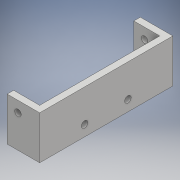
# Autodesk Inventor part: Część2
Saved by Autodesk Inventor 2017 (Build 210142000, 142)
## iProperties
Created: 2019-10-20
Part Number: Część2
Material: Ogólny
Document SubType Name: Modeling
Designer: patry
Density: 1 g/cm^3
Appearance: Domyślna
Author: patry
Autodesk Inventor part; units mm, degrees
ref_plane "YZ Plane" through (0, 0, 0) normal (1, 0, 0) x (0, 1, 0)
ref_plane "XZ Plane" through (0, 0, 0) normal (0, 1, 0) x (-1, 0, 0)
ref_plane "XY Plane" through (0, 0, 0) normal (0, 0, 1) x (1, 0, 0)
sketch "Szkic1" plane through (0, 0, 0) normal (0, 1, 0) x (-1, 0, 0)
  line L0 (7, -35.6103) -> (-8, -35.6103)
  line L1 (-8, -35.6103) -> (-8, -15.6103)
  line L2 (-8, -15.6103) -> (7, -15.6103)
  line L3 (7, -15.6103) -> (7, -35.6103)
  point P0 (0, 0)
  point P1 (2, -20.6103)
  dimension "d21" = 15
  dimension "d22" = 5
  dimension "d23" = 5
  dimension "d24" = 10
  constraints: 8 end point, 2 parallel, 1 horizontal, 1 perpendicular, 1 other
  measures "d21" distance from line of point (2, -20.61) L0
  measures "d22" distance from line of point (2, -20.61) L3
  measures "d23" distance from line of point (2, -20.61) L2
  measures "d24" distance from line of point (2, -20.61) L1
extrude "Wyciągnięcie proste3" add sketch "Szkic1" along normal blind 3
hole "Otwór2" at (-2, 0, -20.6103) direction (0, 1, 0) diameter 3 end through all
sketch "Szkic3" plane through (0, 3, 0) normal (0, 1, 0) x (1, 0, 0)
  line L0 (8, 35.6103) -> (8, 15.6103) projected
  line L1 (8, 35.6103) -> (5, 35.6103)
  line L2 (5, 35.6103) -> (5, 15.6103)
  line L3 (5, 15.6103) -> (8, 15.6103)
  line L4 (8, 15.6103) -> (8, 35.6103)
  point P0 (0, 0)
  dimension "d49" = 3
  constraints: 8 end point, 2 parallel, 1 horizontal, 1 perpendicular
  measures "d49" distance between parallel lines of L2 L0
extrude "Wyciągnięcie proste4" add sketch "Szkic3" along normal blind 55.5
sketch "Szkic4" plane through (0, 58.5, 0) normal (0, 1, 0) x (1, 0, 0)
  line L0 (5, 15.6103) -> (5, 35.6103) projected
  line L1 (5, 35.6103) -> (-7, 35.6103) projected
  line L2 (-7, 35.6103) -> (-7, 15.6103) projected
  line L3 (-7, 15.6103) -> (5, 15.6103) projected
  circle A0 centre (-2, 20.6103) radius 1.5 projected
  line L4 (8, 35.6103) -> (5, 35.6103) projected
  line L5 (5, 35.6103) -> (5, 15.6103) projected
  line L6 (5, 15.6103) -> (8, 15.6103) projected
  line L7 (8, 15.6103) -> (8, 35.6103) projected
  point P0 (0, 0)
extrude "Wyciągnięcie proste5" add sketch "Szkic4" along normal blind 3
sketch "Szkic5" plane through (8, 0, -15.6103) normal (1, 0, 0) x (0, 0, -1)
  line L0 (20, 0) -> (0, 0) projected
  line L1 (20, 0) -> (20, 61.5) projected
  line L2 (0, 61.5) -> (20, 61.5) projected
  line L3 (0, 0) -> (0, 61.5) projected
  point P0 (-15.6103, 0)
  point P1 (15, 40.75)
  point P2 (15, 20.75)
  dimension "d38" = 20
  dimension "d39" = 61.5
  dimension "d40" = 20.75
  dimension "d41" = 5
  measures "d38" distance of point (15, 20.75) point (15, 40.75)
  measures "d39" distance of L0.end L2.start
  measures "d40" distance from line of point (15, 20.75) L0
  measures "d41" distance from line of point (15, 20.75) L1
hole "Otwór3" at (8, 40.75, -30.6103) at (8, 20.75, -30.6103) direction (-1, 0, 0) diameter 3 end through all
equation "\"d22\" = d23"
equation "\"d40\" = 0.5 * d39 - 0.5 * d38"
